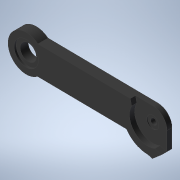
# Autodesk Inventor part: 後ろウィング中間
Saved by Autodesk Inventor 2020.2 (Build 242310000, 310)
## iProperties
Created: 2020-05-05
Part Number: 後ろウィング中間
Material: 一般
Document SubType Name: Modeling
Designer: mozar
Density: 1 g/cm^3
Appearance: 既定
Author: mozar
Autodesk Inventor part; units mm, degrees
ref_plane "YZ Plane" through (0, 0, 0) normal (1, 0, 0) x (0, 1, 0)
ref_plane "XZ Plane" through (0, 0, 0) normal (0, 1, 0) x (-1, 0, 0)
ref_plane "XY Plane" through (0, 0, 0) normal (0, 0, 1) x (1, 0, 0)
sketch "スケッチ1" plane through (0, 0, 0) normal (0, 0, 1) x (1, 0, 0)
  line L0 (-101.5, 48) -> (108.5, 48)
  circle A0 centre (111.885, -19) radius 4
  circle A1 centre (171.8807, -19.7195) radius 4
  circle A2 centre (111.885, -19) radius 7
  circle A3 centre (171.8807, -19.7195) radius 7
  line L1 (171.8807, -19.7195) -> (111.885, -19) construction
  line L2 (171.9647, -12.72) -> (111.969, -12.0005)
  line L3 (111.8011, -25.9995) -> (171.7968, -26.719)
  arc A4 (171.7968, -26.719) -> (171.9647, -12.72) centre (171.8807, -19.7195) ccw
  arc A5 (111.969, -12.0005) -> (111.8011, -25.9995) centre (111.885, -19) ccw
  line L4 (173.7961, -12.9866) -> (250.1906, -34.7195)
  circle A6 centre (241.9819, -63.5746) radius 30
  line L5 (268.18, -78.1916) -> (221.9512, -41.2414)
  line L6 (221.9512, -41.2414) -> (169.9654, -26.4523)
  line L7 (271.9819, -113.1361) -> (271.9819, -54.8199)
  line L8 (111.885, -19) -> (111.885, 41) construction
  line L9 (118.885, -19) -> (118.885, 41)
  line L10 (104.885, 41) -> (104.885, -19)
  arc A7 (104.885, -19) -> (118.885, -19) centre (111.885, -19) ccw
  arc A8 (118.885, 41) -> (104.885, 41) centre (111.885, 41) ccw
  circle A9 centre (29.4318, 47.238) radius 30
  line L11 (113.3193, 34.1485) -> (35.5787, 17.8745)
  line L12 (-0.5585, 48) -> (57.5489, 36.7771)
  line L13 (57.5489, 36.7771) -> (110.4508, 47.8515)
  circle A10 centre (113.5, -20) radius 68
  line L14 (321.9635, -82.9551) -> (60.2705, 100.2843)
  line L15 (259.1892, -39) -> (111.885, -19)
  arc A11 (93.5924, -27.1048) -> (135.371, -5.9244) centre (95.0604, 21.7941) ccw
  arc A12 (135.371, -5.9244) -> (135.8476, -3.6716) centre (132.899, -4.2246) ccw
  arc A13 (135.8476, -3.6716) -> (83.1833, 18.5565) centre (102.1579, -9.9896) ccw
  line L16 (111.885, -19) -> (112.6892, 40.9946) construction
  line L17 (118.8844, -19.0938) -> (119.6886, 40.9008)
  line L18 (105.6898, 41.0884) -> (104.8857, -18.9062)
  arc A14 (104.8857, -18.9062) -> (118.8844, -19.0938) centre (111.885, -19) ccw
  arc A15 (119.6886, 40.9008) -> (105.6898, 41.0884) centre (112.6892, 40.9946) ccw
  line L19 (164.9949, 48) -> (164.9949, 26)
  line L20 (164.9949, 26) -> (327.4949, -102)
  circle A16 centre (116.2926, -40) radius 68
  circle A17 centre (-98.885, 0) radius 67.5
  line L21 (321.3633, -8.501) -> (-152.6681, 78.4982)
  line L22 (104.8897, -3) -> (104.8897, 0)
  line L23 (104.8897, -3) -> (72.0656, -3)
  line L24 (72.0656, 0) -> (104.8897, 0)
  circle A18 centre (83.3769, -17.5) radius 13.85
  line L25 (178.7705, -28.9572) -> (174.2123, -32.8589)
  line L26 (174.2123, -32.8589) -> (164.8807, -30.2042)
  line L27 (164.8807, -30.2042) -> (164.8807, -19.7195)
  line L28 (169.9654, -26.4523) -> (168.5972, -31.2615)
  line L29 (168.5972, -31.2615) -> (164.8807, -26.636)
  line L30 (178.8802, -19.8034) -> (178.6547, -38.6089)
  line L31 (165.0125, -21.0715) -> (158.1724, 13.6763)
  circle A19 centre (171.8807, -19.7195) radius 7.5
  point P0 (0, 0)
  point P1 (141.8829, -19.3597)
  point P2 (111.885, 11)
  point P3 (105.885, 0)
  point P4 (105.885, 0)
  point P5 (23.7328, -42.729)
  point P6 (112.2871, 10.9973)
  point P7 (169.2723, -12.6877)
  point P8 (163.3482, -12.6166)
  point P9 (164.4925, -18.4296)
  point P10 (172.5552, -27.1891)
  point P11 (178.8479, -22.4958)
  dimension "d0" = 8
  dimension "d1" = 8
  dimension "d2" = 3
  dimension "d3" = 3
  dimension "d4" = 60
  dimension "d5" = 14
  dimension "d6" = 14
  dimension "d7" = 60
  dimension "d8" = 14
  dimension "d9" = 60
  dimension "d10" = 14
  dimension "d11" = 6
  dimension "d12" = 35
  dimension "d13" = 13.271
  dimension "d14" = 14
  dimension "d15" = 20
  dimension "d16" = 15
  dimension "d17" = 22
  dimension "d18" = 150
  dimension "d19" = 162.5
  dimension "d20" = 0
  dimension "d21" = 136
  dimension "d22" = 136
  dimension "d23" = 135
  dimension "d24" = 38.227
  dimension "d25" = 18
  dimension "d27" = 5
  dimension "d28" = 6
  dimension "d30" = 101.823
  dimension "d31" = 101.823
  dimension "d32" = 0.5
  constraints: 70 end point, 32 point on circle, 30 tangent, 20 centre point, 7 point on line, 5 vertical, 4 equal length, 4 parallel, 3 coincident, 3 horizontal, 3 midpoint, 2 perpendicular, 1 concentric, 10 other
  measures "d0" diameter of A0
  measures "d1" diameter of A1
  measures "d2" radial gap between concentric circles of A0 A2
  measures "d3" radial gap between concentric circles of A1 A3
  measures "d4" distance of L1.start L1.end
  measures "d5" diameter of A5
  measures "d6" distance from line of L4 L5.end
  measures "d7" diameter of A6
  measures "d8" diameter of A8
  measures "d9" diameter of A9
  measures "d10" distance from line of L11 L12.end
  measures "d11" horizontal distance of L1.end point (105.885, 0)
  measures "d12" angle of L14 L0
  measures "d14" diameter of A15
  measures "d15" vertical distance of L15.start L1.end
  measures "d16" vertical distance of L1.start L4.end
  measures "d17" distance of L19.start L19.end
  measures "d18" vertical distance of L19.start L20.end
  measures "d19" distance from line of L19 L20.end
  measures "d20" distance from line of L19.start L0
  measures "d21" diameter of A10
  measures "d22" diameter of A16
  measures "d23" diameter of A17
  measures "d24" angle of L0 L20
  measures "d25" distance from line of L5.start L20
  measures "d27" distance between parallel lines of L6 L26
  measures "d28" distance of L25.start L25.end
  measures "d30" angle of L11 L8
  measures "d31" angle of L1 L31
  measures "d32" radial gap between concentric circles of A3 A19
extrude "押し出し1" add sketch "スケッチ1" against normal blind 5 contours L25 L26 L28 A19 L15 L6 | L6 L15 L30 | L15 A19 L6 | L6 A19 L30 L15 | A19 L15 L28 L3 L6 | L6 L3 A3 L30 A19 | A19 L28 L15 | L29 L3 L15 A19 L28 | L26 L27 L29 | A2 A11 | L6 A3 L3 | L3 L28 L6 | L28 A19 L15 | L15 A19 L3 L28 | L27 L15 L3 | L3 A2 A11 L15 L27 | A3 | L9 A2 L2 | L2 L17 L9 | L3 A19 L27 L31 A3 L28 | L15 L3 A19 | A2 A11 | L15 L27 A19 L3 | L15 A11 L2 L31 A19 L27 | A19 L31 L2 | L2 A3 L27 L31 A19 | L2 A11 L15 A2 L17 | L31 L27 A3 | A2 L15 A11 | A19 L31 L27 | A0 | A1
extrude "押し出し2" cut sketch "スケッチ1" against normal blind 2.55 contours L6 L15 L30 | L6 A19 L30 L15 | A19 L15 L28 L3 L6 | L6 L3 A3 L30 A19 | A19 L28 L15 | L30 A3 L4 A19 | L6 A3 L3 | L3 L28 L6 | L28 A19 L15 | L15 A19 L3 L28 | A3 | L4 A3 L2 A19 | L3 A19 L27 L31 A3 L28 | A19 L31 L2 | L2 A3 L27 L31 A19 | L31 L27 A3 | A19 L31 L27 | A1
hole "穴1" at (105.885, 0, 0) at (23.7328, -42.729, 0) at (116.2926, -40, 0) at (-98.885, 0, 0) at (171.8807, -19.7195, 0) direction (0, 0, -1) diameter 3 depth 12 tip angle 118
sketch "スケッチ2" plane through (0, 0, 0) normal (0, 0, 1) x (1, 0, 0)
  line L0 (163.3482, -12.6166) -> (164.4925, -18.4296) projected
  arc A0 (164.4925, -18.4296) -> (172.5552, -27.1891) centre (171.8807, -19.7195) ccw projected
  line L1 (172.5552, -27.1891) -> (178.7705, -28.9572) projected
  line L2 (178.7705, -28.9572) -> (174.2123, -32.8589) projected
  line L3 (174.2123, -32.8589) -> (164.8807, -30.2042) projected
  line L4 (164.8807, -30.2042) -> (164.8807, -26.636) projected
  line L5 (164.8807, -26.636) -> (111.8011, -25.9995) projected
  arc A1 (111.969, -12.0005) -> (111.8011, -25.9995) centre (111.885, -19) ccw projected
  line L6 (111.969, -12.0005) -> (163.3482, -12.6166) projected
  circle A2 centre (171.8807, -19.7195) radius 7.5
  circle A3 centre (171.8807, -19.7195) radius 12.5
  point P0 (0, 0)
  point P1 (161.4414, -26.5948)
  point P2 (164.8807, -30.0756)
  point P3 (165.2308, -30.3038)
  point P4 (171.9637, -32.2192)
  dimension "d44" = 5
  constraints: 1 centre point, 1 coincident, 3 other
extrude "押し出し3" add sketch "スケッチ2" against normal blind 5 contours L5 L4 A3 | A3 L3
sketch "スケッチ3" plane through (0, 0, 0) normal (0, 0, 1) x (1, 0, 0)
  line L0 (163.3482, -12.6166) -> (164.4925, -18.4296) projected
  arc A0 (164.4925, -18.4296) -> (172.5552, -27.1891) centre (171.8807, -19.7195) ccw projected
  line L1 (172.5552, -27.1891) -> (178.7705, -28.9572) projected
  line L2 (178.7705, -28.9572) -> (174.2123, -32.8589) projected
  line L3 (174.2123, -32.8589) -> (171.9637, -32.2192) projected
  arc A1 (165.2308, -30.3038) -> (171.9637, -32.2192) centre (171.8807, -19.7195) ccw projected
  line L4 (165.2308, -30.3038) -> (164.8807, -30.2042) projected
  line L5 (164.8807, -30.2042) -> (164.8807, -30.0756) projected
  arc A2 (161.4414, -26.5948) -> (164.8807, -30.0756) centre (171.8807, -19.7195) ccw projected
  line L6 (161.4414, -26.5948) -> (111.8011, -25.9995) projected
  arc A3 (111.969, -12.0005) -> (111.8011, -25.9995) centre (111.885, -19) ccw projected
  line L7 (111.969, -12.0005) -> (163.3482, -12.6166) projected
  circle A4 centre (171.8807, -19.7195) radius 12.5
  point P0 (0, 0)
  point P1 (165.2308, -30.3038)
  constraints: 1 coincident, 3 other
extrude "押し出し4" cut sketch "スケッチ3" against normal blind 10 contours A4 L4 L5
hole "穴2" at (105.885, 0, 0) at (111.885, -19, 0) direction (0, 0, -1) diameter 8.05 depth 12 tip angle 118
sketch "スケッチ4" plane through (0, 0, 0) normal (0, 0, 1) x (1, 0, 0)
  circle A0 centre (111.885, -19) radius 4.025 projected
  line L0 (163.3482, -12.6166) -> (164.4925, -18.4296) projected
  arc A1 (164.4925, -18.4296) -> (172.5552, -27.1891) centre (171.8807, -19.7195) ccw projected
  line L1 (172.5552, -27.1891) -> (178.7705, -28.9572) projected
  line L2 (178.7705, -28.9572) -> (174.2123, -32.8589) projected
  line L3 (174.2123, -32.8589) -> (171.9637, -32.2192) projected
  arc A2 (161.4414, -26.5948) -> (171.9637, -32.2192) centre (171.8807, -19.7195) ccw projected
  line L4 (161.4414, -26.5948) -> (111.8011, -25.9995) projected
  arc A3 (111.969, -12.0005) -> (111.8011, -25.9995) centre (111.885, -19) ccw projected
  line L5 (111.969, -12.0005) -> (163.3482, -12.6166) projected
  arc A4 (164.4925, -18.4296) -> (172.5552, -27.1891) centre (171.8807, -19.7195) ccw projected
  circle A5 centre (171.8807, -19.7195) radius 7.5
  circle A6 centre (171.8807, -19.7195) radius 9
  line L6 (178.7705, -28.9572) -> (172.5552, -27.1891) projected
  line L7 (164.4925, -18.4296) -> (163.3482, -12.6166) projected
  circle A7 centre (111.885, -19) radius 9
  point P0 (0, 0)
  point P1 (175.4063, -28.0002)
  point P2 (163.9203, -15.5231)
  point P3 (163.92, -15.5211)
  point P4 (175.4063, -28.0002)
  dimension "d56" = 15
  dimension "d57" = 1.5
  dimension "d58" = 18
  constraints: 2 coincident, 1 centre point, 1 midpoint, 1 point on line, 6 other
  measures "d58" diameter of A7
extrude "押し出し5" add sketch "スケッチ4" against normal blind 5 contours A7 L4 A3 L5 | L5 A3 L4 A7
extrude "押し出し6" cut sketch "スケッチ4" against normal blind 2.55 contours L0 A1 L1 A6
sketch "スケッチ5" plane through (0, 0, 0) normal (0, 0, 1) x (1, 0, 0)
  arc A0 (117.6254, -12.0683) -> (117.4576, -26.0673) centre (111.885, -19) ccw projected
  line L0 (117.6254, -12.0683) -> (163.3482, -12.6166) projected
  line L1 (163.3482, -12.6166) -> (163.92, -15.5211) projected
  arc A1 (163.92, -15.5211) -> (175.4063, -28.0002) centre (171.8807, -19.7195) ccw projected
  line L2 (175.4063, -28.0002) -> (178.7705, -28.9572) projected
  line L3 (178.7705, -28.9572) -> (174.2123, -32.8589) projected
  line L4 (174.2123, -32.8589) -> (171.9637, -32.2192) projected
  arc A2 (161.4414, -26.5948) -> (171.9637, -32.2192) centre (171.8807, -19.7195) ccw projected
  line L5 (161.4414, -26.5948) -> (117.4576, -26.0673) projected
  circle A3 centre (111.885, -19) radius 4.025 projected
  circle A4 centre (111.885, -19) radius 6
  point P0 (0, 0)
  dimension "d63" = 12
  constraints: 1 centre point, 1 coincident
  measures "d63" diameter of A4
extrude "押し出し7" cut sketch "スケッチ5" against normal blind 1 contours A4
sketch "スケッチ6" plane through (0, 0, 0) normal (0, 0, 1) x (1, 0, 0)
  circle A0 centre (111.885, -19) radius 6 projected
  arc A1 (161.4414, -26.5948) -> (171.9637, -32.2192) centre (171.8807, -19.7195) ccw projected
  line L0 (161.4414, -26.5948) -> (117.4576, -26.0673) projected
  arc A2 (117.6254, -12.0683) -> (117.4576, -26.0673) centre (111.885, -19) ccw projected
  line L1 (117.6254, -12.0683) -> (163.3482, -12.6166) projected
  line L2 (163.3482, -12.6166) -> (163.92, -15.5211) projected
  arc A3 (163.92, -15.5211) -> (175.4063, -28.0002) centre (171.8807, -19.7195) ccw projected
  line L3 (175.4063, -28.0002) -> (178.7705, -28.9572) projected
  line L4 (178.7705, -28.9572) -> (174.2123, -32.8589) projected
  line L5 (174.2123, -32.8589) -> (171.9637, -32.2192) projected
  circle A4 centre (171.8807, -19.7195) radius 1.5 projected
  circle A5 centre (171.8807, -19.7195) radius 3
  point P0 (0, 0)
  dimension "d66" = 6
  constraints: 1 centre point, 1 coincident
  measures "d66" diameter of A5
extrude "押し出し8" cut sketch "スケッチ6" against normal blind 3 contours A5
equation "\"d9\" = d7"
equation "\"d31\" = d30"
